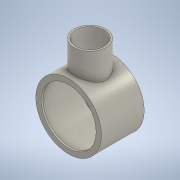
# Autodesk Inventor part: Exhaust
Saved by Autodesk Inventor 2021 (Build 250183000, 183)
## iProperties
Created: 2021-04-23
Part Number: Exhaust
Material: Stainless Steel
Document SubType Name: Modeling
Designer: lucia
Density: 8 g/cm^3
Appearance: Steel - Cast
Author: lucia
Autodesk Inventor part; units mm, degrees
ref_plane "YZ Plane" through (0, 0, 0) normal (1, 0, 0) x (0, 1, 0)
ref_plane "XZ Plane" through (0, 0, 0) normal (0, 1, 0) x (-1, 0, 0)
sketch "Sketch1" plane through (0, 0, 0) normal (0, 0, 1) x (1, 0, 0)
  circle A0 centre (0, 0) radius 14.2875
  circle A1 centre (0, 0) radius 17.4625
  circle A2 centre (0, 0) radius 19.05
  circle A3 centre (0, 0) radius 22.8953
  circle A4 centre (0, 0) radius 24.4828
  circle A5 centre (0, 0) radius 27.6578
  circle A6 centre (0, 0) radius 29.2453
  dimension "d0" = 28.575
  dimension "d1" = 34.925
  dimension "d2" = 38.1
  dimension "d3" = 45.7905
  dimension "d4" = 48.9655
  dimension "d5" = 55.3155
  dimension "d6" = 58.4905
  constraints: 7 centre point, 7 coincident
  measures "d0" diameter of A0
  measures "d1" diameter of A1
  measures "d2" diameter of A2
  measures "d3" diameter of A3
  measures "d4" diameter of A4
  measures "d5" diameter of A5
  measures "d6" diameter of A6
extrude "Extrusion1" add sketch "Sketch1" along normal blind 38.1 contours A0 | A1 | A2 | A3 | A4 | A5 | A6
sketch "Sketch2" plane through (0, 0, 0) normal (0, 1, 0) x (-1, 0, 0)
  circle A0 centre (0, 19.05) radius 14.2875
  line L0 (29.2453, 0) -> (-29.2453, 0) projected
  point P0 (0, 0)
  dimension "d9" = 19.05
  dimension "d10" = 28.575
  constraints: 1 centre point
  measures "d9" distance from line of L0 A0.centre
  measures "d10" diameter of A0
extrude "Extrusion2" add sketch "Sketch2" along normal blind 50.8
shell "Shell1" thickness 1.5875 removed faces 3 at (13.4185, 9.6773, 0) at (13.4185, 9.6773, 38.1) at (-3.9719, 50.8, 19.2449)
sketch "Sketch3" plane through (0, 0, 0) normal (0, 0, 1) x (1, 0, 0)
  circle A0 centre (0, 0) radius 14.2875
  circle A1 centre (0, 0) radius 17.4625
  circle A2 centre (0, 0) radius 19.05
  circle A3 centre (0, 0) radius 22.8953
  circle A4 centre (0, 0) radius 24.4828
  circle A5 centre (0, 0) radius 27.6578
  circle A6 centre (0, 0) radius 29.2453
  dimension "d14" = 28.575
  dimension "d15" = 34.925
  dimension "d16" = 38.1
  dimension "d17" = 45.7905
  dimension "d18" = 48.9655
  dimension "d19" = 55.3155
  dimension "d20" = 58.4905
  constraints: 7 centre point, 7 coincident
  measures "d14" diameter of A0
  measures "d15" diameter of A1
  measures "d16" diameter of A2
  measures "d17" diameter of A3
  measures "d18" diameter of A4
  measures "d19" diameter of A5
  measures "d20" diameter of A6
extrude "Extrusion3" add sketch "Sketch3" along normal blind 1.5875 contours A5
ref_plane "Work Plane1" through (0, 0, 38.1) normal (0, 0, 1) x (1, 0, 0)
sketch "Sketch4" plane through (0, 0, 38.1) normal (0, 0, 1) x (1, 0, 0)
  circle A0 centre (0, 0) radius 14.2875
  circle A1 centre (0, 0) radius 17.4625
  circle A2 centre (0, 0) radius 19.05
  circle A3 centre (0, 0) radius 22.8953
  circle A4 centre (0, 0) radius 24.4828
  circle A5 centre (0, 0) radius 27.6578
  circle A6 centre (0, 0) radius 29.2453
  dimension "d24" = 28.575
  dimension "d25" = 34.925
  dimension "d26" = 38.1
  dimension "d27" = 45.7905
  dimension "d28" = 48.9655
  dimension "d29" = 55.3155
  dimension "d30" = 58.4905
  constraints: 7 centre point, 7 coincident
  measures "d24" diameter of A0
  measures "d25" diameter of A1
  measures "d26" diameter of A2
  measures "d27" diameter of A3
  measures "d28" diameter of A4
  measures "d29" diameter of A5
  measures "d30" diameter of A6
extrude "Extrusion4" add sketch "Sketch4" against normal blind 1.5875 contours A5
body "Solid1"
